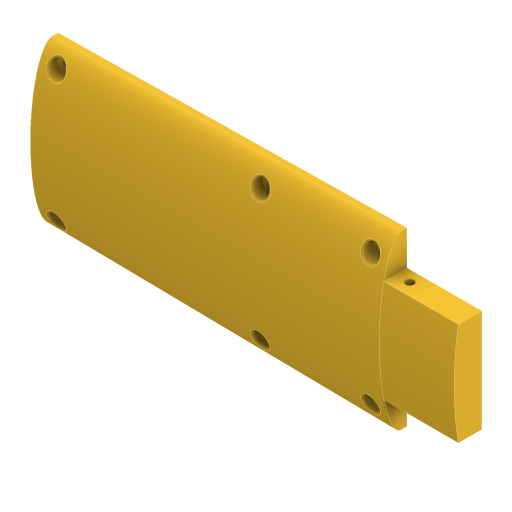
# Autodesk Inventor part: BodyStructure Side
Saved by Autodesk Inventor 2023 (Build 270158000, 158)
## iProperties
Created: 2022-01-14
Part Number: BodyStructure Side
Material: Generic
Document SubType Name: Modeling
Designer: Jochen
Density: 1 g/cm^3
Appearance: Default
Author: Jochen
Autodesk Inventor part; units mm, degrees
ref_plane "YZ Plane" through (0, 0, 0) normal (1, 0, 0) x (0, 1, 0)
ref_plane "Work Plane1" through (0, 0, 50) normal (0, 0, 1) x (1, 0, 0)
sketch "Sketch1" plane through (0, 0, 50) normal (0, 0, 1) x (1, 0, 0)
  line L0 (0, -18.5) -> (0, 18.5)
  line L1 (0, 18.5) -> (-9, 18.5)
  line L2 (-9, -31) -> (-135, -29)
  line L3 (-135, -29) -> (-135, 29)
  line L4 (-135, 29) -> (-9, 31)
  line L5 (-9, 31) -> (-9, 18.5)
  line L6 (-9, -18.5) -> (0, -18.5)
  line L7 (0, -50.4497) -> (0, 50.4497) construction
  line L8 (-165.6, 0) -> (48.6, 0) construction
  line L9 (-9, -18.5) -> (-9, -31)
  line L10 (0, -18.5) -> (18, -18.5)
  line L11 (18, -18.5) -> (18, 18.5)
  line L12 (18, 18.5) -> (0, 18.5)
  point P0 (0, 0)
  point P1 (-9, -24.75)
  dimension "d2" = 135
  dimension "d3" = 37
  dimension "d4" = 9
  dimension "d7" = 58
  dimension "d73" = 126
  dimension "d99" = 18
  dimension "d114" = 62
  constraints: 22 end point, 5 perpendicular, 3 point on line, 1 horizontal, 1 midpoint, 1 parallel, 1 vertical, 3 other
  measures "d2" distance between parallel lines of L3 L7
  measures "d3" distance of L0.start L0.end
  measures "d4" distance between parallel lines of L7 L9
  measures "d7" distance of L2.end L3.end
  measures "d73" distance from line of L3 point (-9, -24.75)
  measures "d99" distance of L0.start L10.end
  measures "d114" distance of L4.end L2.start
extrude "Extrusion1" add sketch "Sketch1" along normal blind 10
sketch "Sketch8" plane through (-135, -29, 50) normal (-1, 0, 0) x (0, 0, 1)
  line L0 (0, 0) -> (10, 0) projected
  line L1 (0, 58) -> (0, 0) projected
  line L2 (0, 0) -> (10, 0) projected
  line L3 (10, 58) -> (10, 0) construction
  line L4 (0, 58) -> (10, 58) projected
  line L5 (2, 58) -> (2, 0) construction
  line L6 (10, 58) -> (10, 0) construction
  line L7 (2, 58) -> (0, 58)
  line L8 (0, 0) -> (2, 0)
  line L9 (0, 58) -> (0, 0)
  ellipse E0 centre (2, 29) end of major axis (2, 58) minor radius 8 (2, 0) -> (2, 58) ccw
  point P0 (-50, 29)
  dimension "d144" = 8
  constraints: 10 end point, 4 point on line, 2 perpendicular, 1 collinear, 1 horizontal, 1 parallel, 1 vertical, 4 other
  measures "d144" distance between parallel lines of L5 L3
sketch "Sketch11" plane through (-9, -32.1471, 50) normal (1, 0, 0) x (0, 0, -1)
  line L0 (0, 63.1471) -> (-10, 63.1471)
  line L1 (-10, 34.7458) -> (-10, 63.1471) construction
  line L2 (-9, 1.1471) -> (-9, 1.5)
  line L3 (0, 1.1471) -> (-9, 1.1471)
  line L4 (-2, 63.1471) -> (-2, 1.1471) construction
  line L5 (-2, 63.1471) -> (0, 63.1471)
  line L6 (0, 63.1471) -> (0, 1.1471)
  line L7 (0, 1.1471) -> (-2, 1.1471)
  line L8 (-10, 13.6471) -> (-10, 50.6471) projected
  ellipse E0 centre (-2, 32.1471) end of major axis (-2, 63.1471) minor radius 8 (-2, 63.1471) -> (-2, 1.1471) ccw
  point P0 (50, 30.6471)
  point P1 (0, 20.1358)
  dimension "d145" = 8
  constraints: 16 end point, 3 perpendicular, 3 point on line, 1 horizontal, 1 vertical, 4 other
  measures "d145" distance between parallel lines of L4 L1
sketch "Sketch9" plane through (18, 21.5, 50) normal (1, 0, 0) x (0, 0, -1)
  line L0 (0, -3) -> (0, 9.5) projected
  line L1 (-10, -3) -> (-10, 9.5) construction
  line L2 (0, -40) -> (0, 0) projected
  line L3 (0, -52.5) -> (0, -40) projected
  line L4 (-10, -52.5) -> (-10, -40) construction
  line L5 (-2, 9.5) -> (-2, -52.5) construction
  line L6 (-2, 9.5) -> (0, 9.5)
  line L7 (0, 9.5) -> (0, -52.5)
  line L8 (0, -52.5) -> (-2, -52.5)
  ellipse E0 centre (-2, -21.5) end of major axis (-2, 9.5) minor radius 8 (-2, 9.5) -> (-2, -52.5) ccw
  point P0 (50, -21.5)
  dimension "d146" = 8
  constraints: 8 end point, 2 perpendicular, 1 horizontal, 1 vertical, 4 other
  measures "d146" distance between parallel lines of L4 L5
loft "Loft4" add profiles "Sketch11", "Sketch9" separate body
loft "Loft5" add profiles "Sketch11", "Sketch8" bodies 2
combine bodies "Combine1" operation type common bodies to combine 1 2
sketch "Sketch2" plane through (0, 0, 50) normal (0, 0, 1) x (1, 0, 0)
  circle A0 centre (-55, -23.5) radius 1.5
  circle A1 centre (-15, -23.5) radius 1.5
  circle A2 centre (-55, 23.5) radius 1.5
  circle A3 centre (-15, 23.5) radius 1.5
  line L0 (-135, -11) -> (-127, -11)
  line L1 (-125, -9) -> (-125, 9)
  line L2 (-127, 11) -> (-135, 11)
  line L3 (-135, 11) -> (-135, -11)
  arc A4 (-127, -11) -> (-125, -9) centre (-127, -9) ccw
  arc A5 (-125, 9) -> (-127, 11) centre (-127, 9) ccw
  line L4 (18, -18.5) -> (-9, -18.5) projected
  line L5 (-9, -18.5) -> (-9, -31) projected
  line L6 (-135, -29) -> (-135, 29) projected
  line L7 (-9, 31) -> (-9, 18.5) projected
  line L8 (18, -18.5) -> (-9, -18.5) projected
  line L9 (-9, -18.5) -> (-9, -31) projected
  line L10 (-9, 31) -> (-9, 18.5) projected
  line L11 (0, -50.4497) -> (0, 50.4497) construction
  line L12 (-165.6, 0) -> (48.6, 0) construction
  line L13 (-135, 29) -> (-135, -29) construction
  arc A6 (-52, -23.5) -> (-58, -23.5) centre (-55, -23.5) ccw
  arc A7 (-12, -23.5) -> (-18, -23.5) centre (-15, -23.5) ccw
  arc A8 (-58, 23.5) -> (-52, 23.5) centre (-55, 23.5) ccw
  arc A9 (-18, 23.5) -> (-12, 23.5) centre (-15, 23.5) ccw
  line L14 (-7.75, -17) -> (-7.75, 17)
  line L15 (-19.5, 23.5) -> (-50.5, 23.5)
  line L16 (-54, 19.1125) -> (-54, -19.1125)
  line L17 (-50.5, -23.5) -> (-19.5, -23.5)
  line L18 (-55, -23.5) -> (-55, 23.5) construction
  line L19 (-56, -19.1125) -> (-56, 19.1125)
  arc A10 (-50.5, -23.5) -> (-54, -19.1125) centre (-55, -23.5) ccw
  arc A11 (-89.9151, 22.0406) -> (-89.9151, 22.0406) centre (-89.5655, 22.4764) ccw
  line L20 (-123, 22.5184) -> (-123, -22.4816)
  line L21 (-58, -23.5) -> (-58, -30.2222)
  line L22 (-52, -23.5) -> (-52, -30.3175)
  line L23 (-135, -29) -> (-9, -31) projected
  line L24 (-18, -23.5) -> (-18, -31)
  line L25 (-12, -23.5) -> (-12, -30.9524)
  line L26 (-12, 23.5) -> (-12, 30.9524)
  line L27 (-18, 23.5) -> (-18, 30.8571)
  line L28 (-52, 23.5) -> (-52, 30.3175)
  line L29 (-58, 23.5) -> (-58, 30.2222)
  line L30 (-9, 31) -> (-135, 29) projected
  line L31 (-135, -29) -> (-135, 29) projected
  arc A12 (-49.3875, 23.2839) -> (-49.3875, 23.2839) centre (-49.8289, 22.9413) ccw
  arc A13 (-56, -19.1125) -> (-59.4994, -23.4278) centre (-55, -23.5) ccw
  arc A14 (-59.5, 23.5) -> (-56, 19.1125) centre (-55, 23.5) ccw
  arc A15 (-54, 19.1125) -> (-50.5, 23.5) centre (-55, 23.5) ccw
  arc A16 (-9, 19) -> (-9, 19) centre (-9, 20) ccw
  line L32 (-50.5, 23.5) -> (-50.5, 23.5)
  line L33 (-59.5, 23.5) -> (-59.5, 23.5)
  line L34 (-123, -22.4816) -> (-59.5006, -23.5)
  line L35 (-59.5, 23.5) -> (-123, 22.5184)
  line L36 (-59.4994, -23.4278) -> (-59.5006, -23.5)
  line L37 (-50.5, -23.5) -> (-50.5, -23.5)
  circle A17 centre (-129, -23.5) radius 1.5
  arc A18 (-126, -23.5) -> (-132, -23.5) centre (-129, -23.5) ccw
  line L38 (-126, -23.5) -> (-126, -29.1429)
  line L39 (-132, -23.5) -> (-132, -29.0392)
  circle A19 centre (-129, 23.5) radius 1.5
  arc A20 (-132, 23.5) -> (-126, 23.5) centre (-129, 23.5) ccw
  line L40 (-126, 23.5) -> (-126, 29.1429)
  line L41 (-132, 23.5) -> (-132, 29.0392)
  line L42 (-15, 23.5) -> (-129, 23.5) construction
  arc A21 (-126, 23.5) -> (-132, 23.5) centre (-129, 23.5) ccw
  arc A22 (-52, 23.5) -> (-58, 23.5) centre (-55, 23.5) ccw
  arc A23 (-12, 23.5) -> (-18, 23.5) centre (-15, 23.5) ccw
  arc A24 (-132, -23.5) -> (-126, -23.5) centre (-129, -23.5) ccw
  arc A25 (-58, -23.5) -> (-52, -23.5) centre (-55, -23.5) ccw
  arc A26 (-18, -23.5) -> (-12, -23.5) centre (-15, -23.5) ccw
  line L43 (0, -17) -> (0, 17)
  line L44 (0, 17) -> (17, 17)
  line L45 (17, 17) -> (17, -17)
  line L46 (17, -17) -> (0, -17)
  line L47 (18, -18.5) -> (18, 18.5) construction
  line L48 (0, -18.5) -> (18, -18.5) construction
  line L49 (18, 18.5) -> (0, 18.5) construction
  line L50 (-4, -12.5) -> (-4, 12.5) construction
  line L51 (-2.25, -12.5) -> (-2.25, 12.5)
  line L52 (-5.75, 12.5) -> (-5.75, -12.5)
  arc A27 (-5.75, -12.5) -> (-2.25, -12.5) centre (-4, -12.5) ccw
  arc A28 (-2.25, 12.5) -> (-5.75, 12.5) centre (-4, 12.5) ccw
  line L53 (18, 18.5) -> (18, -18.5) projected
  line L54 (-9, 18.5) -> (18, 18.5) projected
  line L55 (18, 18.5) -> (18, -18.5) projected
  line L56 (-9, 18.5) -> (18, 18.5) projected
  line L57 (-135, 29) -> (-9, 31) projected
  line L58 (-9, -31) -> (-135, -29) projected
  line L59 (-135, 29) -> (-9, 31) projected
  line L60 (-9, -31) -> (-135, -29) projected
  line L61 (-7.75, 17) -> (-10.5, 17)
  line L62 (-7.75, -17) -> (-10.8407, -17)
  line L63 (-19.5, 23.5) -> (-19.5, 21)
  arc A29 (-19.5, 21) -> (-15.5, 17) centre (-15.5, 21) ccw
  line L64 (-15.5, 17) -> (-10.5, 17)
  line L65 (-19.5, -23.5) -> (-19.5, -21)
  arc A30 (-15.5, -17) -> (-19.5, -21) centre (-15.5, -21) ccw
  line L66 (-15.5, -17) -> (-10.8407, -17)
  point P0 (0, 0)
  point P1 (-2.5, 0)
  point P2 (-33.565, -30.9847)
  point P3 (-135, 0)
  point P4 (-54.5017, 19)
  point P5 (-50.7819, 25.4474)
  point P6 (-4, 0)
  dimension "d12" = 2
  dimension "d13" = 22
  dimension "d14" = 10
  dimension "d15" = 3
  dimension "d16" = 6
  dimension "d17" = 47
  dimension "d18" = 47
  dimension "d21" = 15
  dimension "d29" = 2
  dimension "d30" = 2
  dimension "d77" = 1.5
  dimension "d91" = 6
  dimension "d102" = 55
  dimension "d104" = 1
  dimension "d105" = 0
  dimension "d110" = 25
  dimension "d111" = 3.5
  dimension "d112" = 5
  dimension "d113" = 2
  dimension "d131" = 45
  dimension "d147" = 1.5
  dimension "d149" = 4
  dimension "d150" = 1.5
  constraints: 90 end point, 50 point on circle, 31 centre point, 29 tangent, 18 equal radius, 15 vertical, 12 point on line, 10 coincident, 8 perpendicular, 7 collinear, 6 parallel, 5 horizontal, 3 equal length, 3 midpoint, 2 symmetric about line, 8 other
  measures "d12" radius of A4
  measures "d13" distance of L2.end L0.start
  measures "d14" distance between parallel lines of L6 L1
  measures "d15" diameter of A1
  measures "d16" diameter of A7
  measures "d17" distance of A2.centre A0.centre
  measures "d18" distance of A3.centre A1.centre
  measures "d21" distance from line of L11 A1.centre
  measures "d29" distance between parallel lines of L16 L19
  measures "d30" distance between parallel lines of L20 L1
  measures "d77" radial gap between concentric circles of A15 A8
  measures "d91" distance from line of L31 A17.centre
  measures "d102" distance between parallel lines of L11 L18
  measures "d104" distance from line of L4.start L45
  measures "d105" distance from line of L11 L43.start
  measures "d110" distance of L50.start L50.end
  measures "d111" diameter of A28
  measures "d112" distance between parallel lines of L50 L5
  measures "d113" distance between parallel lines of L14 L52
  measures "d131" distance of L20.start L20.end
  measures "d149" radius of A29
  measures "d150" distance from line of L15.start L27
extrude "Extrusion2" cut sketch "Sketch2" along normal blind 5 contours A0 | A1 | A2 | A3 | L3 L2 A5 L1 A4 L0 | A12 | L62 L66 A30 L65 L17 A10 L16 A15 L15 L63 A29 L64 L61 L14 | A11 | A13 L36 L34 L20 L35 A14 L19 | A17 | A19 | L43 L44 L45 L46 | A27 L52 A28 L51 bodies 1
sketch "Sketch3" plane through (0, 0, 0) normal (1, 0, 0) x (0, 1, 0)
  line L0 (0, -12.1645) -> (0, 72.9869) construction
  line L1 (-50.4497, 0) -> (50.4497, 0) construction
  line L2 (-31, 50.5602) -> (-20, 50.5602) construction
  line L3 (-20, 50) -> (-20, 60) construction
  line L4 (20, 50) -> (31, 50) construction
  line L5 (-31, 50) -> (-31, 54)
  line L6 (-26, 59) -> (26, 59)
  line L7 (31, 50) -> (20, 50) projected
  line L8 (31, 50) -> (-31, 50)
  line L9 (31, 54) -> (31, 50)
  line L10 (18.5, 50) -> (31, 50) construction
  line L11 (-20, 50) -> (20, 50) construction
  line L12 (20, 50) -> (20, 56.9796) construction
  line L13 (-20, 50) -> (-20, 56.9796) construction
  line L14 (-31, 50) -> (-18.5, 50) construction
  arc A0 (-26, 59) -> (-31, 54) centre (-26, 54) ccw
  arc A1 (31, 54) -> (26, 59) centre (26, 54) ccw
  line L15 (-31, 50.5) -> (31, 50.5)
  line L16 (-18.5, 50) -> (-18.5, 58.4193) projected
  line L17 (18.5, 50) -> (18.5, 58.4193) projected
  line L18 (18.5, 58.4193) -> (18.5, 50) projected
  line L19 (-18.5, 50) -> (-18.5, 58.4193) projected
  line L20 (18.5, 58.4193) -> (18.5, 50) projected
  line L21 (-18.5, 50) -> (-18.5, 58.4193) projected
  line L22 (-31, 50) -> (-31, 52) projected
  line L23 (31, 50) -> (31, 52) projected
  line L24 (18.5, 50) -> (17, 50) projected
  line L25 (17, 50) -> (17, 55) projected
  line L26 (17, 55) -> (-17, 55) projected
  line L27 (-17, 55) -> (-17, 50) projected
  line L28 (17, 50) -> (-17, 50) projected
  line L29 (-17, 50) -> (-18.5, 50) projected
  line L30 (18.5, 50) -> (17, 50) projected
  line L31 (17, 50) -> (17, 55) projected
  line L32 (17, 55) -> (-17, 55) projected
  line L33 (-17, 55) -> (-17, 50) projected
  line L34 (17, 50) -> (-17, 50) projected
  line L35 (-17, 50) -> (-18.5, 50) projected
  ellipse E0 centre (0, 52) end of major axis (31, 52) minor radius 8 (18.5, 58.4193) -> (-18.5, 58.4193) ccw projected
  ellipse E1 centre (0, 52) end of major axis (31, 52) minor radius 8 (18.5, 58.4193) -> (-18.5, 58.4193) ccw projected
  point P0 (0, 0)
  point P1 (27, 55.9779)
  point P2 (-20, 56.9789)
  point P3 (20, 56.9789)
  point P4 (19, 50)
  point P5 (-19, 50)
  dimension "d65" = 0.5
  dimension "d92" = 5
  constraints: 12 end point, 4 point on circle, 2 centre point, 2 tangent, 1 coincident, 1 horizontal, 1 parallel, 1 point on line, 11 other
  measures "d65" distance between parallel lines of L8 L15
  measures "d92" radius of A1
extrude "Extrusion10" [suppressed]
ref_plane "Work Plane2" through (0, 0, 60) normal (0, 0, -1) x (-1, 0, 0)
extrude "Extrusion11" cut sketch "Sketch2" against normal blind 7 from surface at 10 contours A0 | A1 | A2 | A3 | A6 A25 | A22 A8 | A7 A26 | A23 A9 | A17 | A24 A18 | A19 | A21 A20 bodies 1
extrude "Extrusion6" cut sketch "Sketch2" along normal through all contours A0 | A1 | A2 | A3 bodies 1
sketch "Sketch4" plane through (0, 0, 0) normal (0, 1, 0) x (-1, 0, 0)
  line L0 (0, -12.1645) -> (0, 72.9869) construction
  line L1 (14.4, 0) -> (-23.4, 0) construction
  circle A0 centre (4, 54) radius 1.5
  line L2 (9, 50) -> (-18, 50) construction
  line L3 (9, 59) -> (-18, 59) construction
  point P0 (0, 0)
  point P1 (4, 50)
  point P2 (0, 50)
  point P3 (9, 60)
  point P4 (0, 59)
  point P5 (5.5, 50.5)
  point P6 (7, 60)
  point P7 (-17, 50)
  dimension "d52" = 3
  dimension "d66" = 5
  dimension "d115" = 4
  constraints: 1 centre point, 1 other
  measures "d52" diameter of A0
  measures "d115" distance from line of L0 A0.centre
extrude "Extrusion7" cut sketch "Sketch4" along normal through all both and the other way through all bodies 1
sketch "Sketch5" plane through (0, 0, 0) normal (1, 0, 0) x (0, 1, 0)
  circle A0 centre (15, 54) radius 1.5
  circle A1 centre (-15, 54) radius 1.5
  line L0 (-19, 50) -> (19, 50) projected
  line L1 (0, -12.1645) -> (0, 72.9869) construction
  line L2 (-50.4497, 0) -> (50.4497, 0) construction
  line L3 (-20, 59) -> (20, 59) construction
  point P0 (0, 0)
  point P1 (-17, 50)
  point P2 (17, 50)
  dimension "d56" = 3
  dimension "d58" = 30
  dimension "d67" = 5
  constraints: 2 centre point, 1 equal radius, 1 symmetric about line
  measures "d56" diameter of A1
  measures "d58" distance of A0.centre A1.centre
  measures "d67" distance from line of L3 A0.centre
extrude "Extrusion8" cut sketch "Sketch5" along normal blind 10 from surface at -135 bodies 1
fillet "Fillet2" radius 2 2 edges at (-7.75, 17, 52.5) (-7.75, -17, 52.5)
fillet "Fillet2" radius 1 17 edges at (-35, 23.5, 55) (-51.4822, 20.6938, 55) (-54, 0, 55) (-123, 0.0184, 55) (-91.25, 23.0092, 55) (-58.5178, 20.6938, 55) (-7.75, 0, 55) (-35, -23.5, 55) (-51.4822, -20.6938, 55) (-58.4952, -20.6656, 55) (-56, 0, 55) (-54, 19.1125, 52.5) (-56, 19.1125, 52.5) (-56, -19.1125, 52.5) (-54, -19.1125, 52.5) (-19.5, -23.5, 52.5) (-59.5, 23.5, 52.5)
fillet "Fillet3" radius 0.5 13 edges at (-12.2953, 22.2021, 57.5732) (-17.681, 24.8462, 56.7454) (-52.7817, 21.4803, 57.6433) (-57.1846, 25.5561, 56.2751) (-12.1785, -22.4807, 57.4985) (-17.793, -24.5951, 56.8321) (-53.7803, -20.7591, 57.8256) (-56.209, -26.2456, 55.978) (-126.8319, -21.4265, 57.4197) (-128.9993, -26.5, 55.3028) (-131.1837, -21.443, 57.3995) (-126.8005, 21.4598, 57.4099) (-131.1508, 25.5915, 55.7907)
equation "\"d18\" = d17"
body "Solid1"
